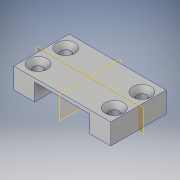
# Autodesk Inventor part: mounting channel
Saved by Autodesk Inventor 2018 (Build 220112000, 112)
## iProperties
Created: 2018-02-15
Part Number: mounting channel
Material: Aluminum 6061
Document SubType Name: Modeling
Designer: licajohn
Density: 2.7 g/cm^3
Appearance: Aluminum - Flat
Mass: 20.0613 g
Surface Area: 39.5573 cm^2
Volume: 7.43013 cm^3
Author: licajohn
Autodesk Inventor part; units mm, degrees
ref_plane "YZ Plane" through (0, 0, 0) normal (1, 0, 0) x (0, 1, 0)
ref_plane "XZ Plane" through (0, 0, 0) normal (0, 1, 0) x (-1, 0, 0)
ref_plane "XY Plane" through (0, 0, 0) normal (0, 0, 1) x (1, 0, 0)
sketch "Sketch1" plane through (0, 0, 0) normal (0, 0, 1) x (1, 0, 0)
  line L0 (0, 0) -> (44.45, 0)
  line L1 (44.45, 0) -> (44.45, 9.525)
  line L2 (44.45, 9.525) -> (0, 9.525)
  line L3 (0, 9.525) -> (0, 0)
  line L4 (9.525, 0) -> (34.925, 0)
  line L5 (34.925, 0) -> (34.925, 7.9375)
  line L6 (34.925, 7.9375) -> (9.525, 7.9375)
  line L7 (9.525, 7.9375) -> (9.525, 0)
  line L8 (22.225, 9.525) -> (22.225, 0) construction
  dimension "d0" = 44.45
  dimension "d1" = 9.525
  dimension "d2" = 7.9375
  dimension "d3" = 25.4
  dimension "d4" = 9.525
  dimension "d5" = 9.525
  constraints: 18 end point, 4 parallel, 2 horizontal, 2 midpoint, 2 perpendicular, 1 point on line, 1 vertical
  measures "d0" distance of L2.end L1.end
  measures "d1" distance of L0.end L1.end
  measures "d2" distance of L4.end L5.end
  measures "d3" distance between parallel lines of L7 L5
  measures "d4" distance between parallel lines of L1 L5
  measures "d5" distance between parallel lines of L3 L7
extrude "Extrusion1" add sketch "Sketch1" along normal blind 25.4 contours L3 L2 L1 L0 L5 L6 L7
sketch "Sketch2" plane through (0, 0, 0) normal (0, -1, 0) x (1, 0, 0)
  line L0 (9.525, 0) -> (9.525, 25.4) projected
  line L1 (0, 25.4) -> (9.525, 25.4) projected
  line L2 (0, 0) -> (0, 25.4) projected
  line L3 (0, 0) -> (9.525, 0) projected
  line L4 (34.925, 25.4) -> (34.925, 0) projected
  line L5 (34.925, 0) -> (44.45, 0) projected
  line L6 (44.45, 0) -> (44.45, 25.4) projected
  line L7 (34.925, 25.4) -> (44.45, 25.4) projected
  point P0 (4.7625, 19.05)
  point P1 (4.7625, 6.35)
  point P2 (39.6875, 6.35)
  point P3 (39.6875, 19.05)
  dimension "d8" = 12.7
  dimension "d9" = 6.35
  dimension "d10" = 6.35
  dimension "d12" = 34.925
  dimension "d13" = 34.925
  dimension "d14" = 44.45
  dimension "d15" = 4.7625
  constraints: 2 horizontal alignment
  measures "d8" distance of point (4.762, 6.35) point (4.762, 19.05)
  measures "d9" distance from line of L1 point (4.762, 19.05)
  measures "d10" distance from line of L3 point (4.762, 6.35)
  measures "d12" distance of point (39.688, 19.05) point (4.762, 19.05)
  measures "d13" distance of point (4.762, 6.35) point (39.687, 6.35)
  measures "d14" distance between parallel lines of L6 L2
  measures "d15" distance from line of L6 point (39.688, 19.05)
sketch "Sketch3" plane through (0, 9.525, 0) normal (0, 1, 0) x (1, 0, 0)
  point P0 (0, 0)
  point P1 (4.7625, -19.05)
  point P2 (4.7625, -6.35)
  point P3 (39.6875, -6.35)
  point P4 (39.6875, -19.05)
hole "Hole1" at (39.6875, 9.525, 19.05) at (39.6875, 9.525, 6.35) at (4.7625, 9.525, 19.05) at (4.7625, 9.525, 6.35) direction (0, -1, 0) diameter 4.4958 end through all countersink diameter 8.4328 countersink angle 82
ref_plane "Work Plane1" through (22.225, 0, 0) normal (1, 0, 0) x (0, 0, -1)
ref_plane "Work Plane2" through (0, 0, 12.7) normal (0, 0, 1) x (1, 0, 0)
equation "\"d13\" = d12"
equation "\"d15\" = -0.5 * d12 + 0.5 * d14"
body "Solid1"
